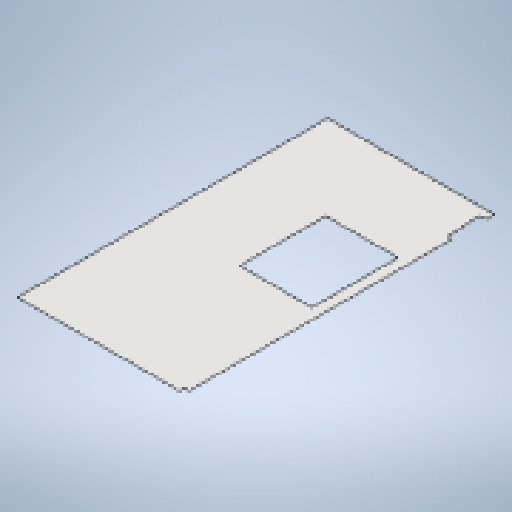
# Autodesk Inventor part: PNS-0111 floor sheet 2
Saved by Autodesk Inventor 2025.1 (Build 291241020, 241B)
## iProperties
Created: 2025-03-10
Part Number: PNS-0111 floor sheet 2
Material: Stainless Steel
Document SubType Name: Sheet Metal
Designer: user
Stock Number: PNS-0111 floor sheet 2
Mass: 72000 g
Surface Area: 90180 cm^2
Volume: 9000 cm^3
Density: 8 g/cm^3
Sheet Metal Rule: AISI304 2mm Die16
Sheet Metal Width: 1385.000 mm
Sheet Metal Length: 2575.000 mm
Sheet Metal Area: 3566375.000 mm^2
Appearance: Default
Flat Pattern Width: 138.5 cm
Flat Pattern Length: 257.5 cm
Flat Pattern Area: 35663.7 cm^2
Author: admin
Autodesk Inventor part; units mm, degrees
ref_plane "YZ Plane" through (0, 0, 0) normal (1, 0, 0) x (0, 1, 0)
ref_plane "XZ Plane" through (0, 0, 0) normal (0, 1, 0) x (-1, 0, 0)
ref_plane "XY Plane" through (0, 0, 0) normal (0, 0, 1) x (1, 0, 0)
sketch "Sketch1" plane through (0, 0, 0) normal (0, 0, 1) x (1, 0, 0)
  line L0 (-692.5, -1287.5) -> (692.5, -1287.5)
  line L1 (692.5, -1287.5) -> (692.5, 1287.5)
  line L2 (692.5, 1287.5) -> (-692.5, 1287.5)
  line L3 (-692.5, 1287.5) -> (-692.5, -1287.5)
  line L4 (-692.5, -1287.5) -> (692.5, 1287.5) construction
  line L5 (692.5, -1287.5) -> (-692.5, 1287.5) construction
  line L6 (692.5, -1247.5) -> (652.5, -1247.5)
  line L7 (652.5, -1247.5) -> (652.5, -1287.5)
  line L8 (692.5, 1222.5) -> (652.5, 1222.5)
  line L9 (652.5, 1222.5) -> (652.5, 932.5)
  line L10 (652.5, 932.5) -> (692.5, 932.5)
  line L11 (692.5, 932.5) -> (692.5, 1222.5)
  line L12 (652.5, 1067.5) -> (642.5, 1067.5)
  line L13 (642.5, 1067.5) -> (642.5, 1217.5)
  line L14 (642.5, 1217.5) -> (652.5, 1217.5)
  line L15 (-572.5, -767.5) -> (17.5, -767.5)
  line L16 (17.5, -767.5) -> (17.5, -177.5)
  line L17 (17.5, -177.5) -> (-572.5, -177.5)
  line L18 (-572.5, -177.5) -> (-572.5, -767.5)
  point P0 (0, 0)
  dimension "d154" = 1385
  dimension "d155" = 2575
  dimension "d157" = 40
  dimension "d159" = 290
  dimension "d161" = 40
  dimension "d162" = 2220
  dimension "d163" = 10
  dimension "d164" = 150
  dimension "d165" = 5
  dimension "d166" = 590
  dimension "d167" = 590
  dimension "d168" = 675
  dimension "d169" = 520
  measures "d154" distance of L1.end L2.end
  measures "d155" distance of L0.end L1.end
  measures "d157" distance of L6.start L6.end
  measures "d159" distance of L8.end L9.end
  measures "d161" distance of L9.end L10.end
  measures "d162" distance between parallel lines of L10 L0
  measures "d163" distance of L12.start L12.end
  measures "d164" distance of L12.end L13.end
  measures "d165" distance between parallel lines of L8 L14
  measures "d166" distance of L17.end L15.start
  measures "d167" distance of L16.end L17.end
  measures "d168" distance between parallel lines of L16 L1
  measures "d169" distance between parallel lines of L15 L0
extrude "Plate5" add sketch "Sketch1" along normal blind 2 contours L3 L2 L1 L8 L9 L14 L13 L12 L10 L6 L7 L0
fillet "Corner Round1" radius 15 1 edges at (652.5, -1247.5, 1)
body "Solid3"
